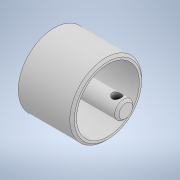
# Autodesk Inventor part: Part4
Saved by Autodesk Inventor 2021 (Build 250183000, 183)
## iProperties
Created: 2021-03-30
Part Number: Part4
Material: Generic
Document SubType Name: Modeling
Designer: Ariel Wolle
Density: 1 g/cm^3
Appearance: Default
Author: Ariel Wolle
Autodesk Inventor part; units mm, degrees
ref_plane "YZ Plane" through (0, 0, 0) normal (1, 0, 0) x (0, 1, 0)
ref_plane "XZ Plane" through (0, 0, 0) normal (0, 1, 0) x (-1, 0, 0)
ref_plane "XY Plane" through (0, 0, 0) normal (0, 0, 1) x (1, 0, 0)
sketch "Sketch1" plane through (0, 0, 0) normal (1, 0, 0) x (0, 1, 0)
  circle A0 centre (0, 0) radius 12.7
  dimension "d0" = 25.4
  constraints: 1 centre point, 1 coincident
  measures "d0" diameter of A0
extrude "Extrusion1" add sketch "Sketch1" along normal blind 19.05
sketch "Sketch2" plane through (19.05, 0, 0) normal (1, 0, 0) x (0, 0, -1)
  circle A0 centre (0, 0) radius 11.1125
  dimension "d3" = 22.225
  constraints: 1 centre point, 1 coincident
  measures "d3" diameter of A0
extrude "Extrusion2" cut sketch "Sketch2" against normal blind 15.875
sketch "Sketch3" plane through (3.175, 0, 0) normal (1, 0, 0) x (0, 0, -1)
  circle A0 centre (0, 0) radius 3.175
  dimension "d6" = 6.35
  constraints: 1 centre point, 1 coincident
  measures "d6" diameter of A0
extrude "Extrusion3" add sketch "Sketch3" along normal blind 22.225
sketch "Sketch4" plane through (0, 0, 0) normal (0, 1, 0) x (-1, 0, 0)
  circle A0 centre (-22.225, 0) radius 1.5875
  line L0 (-25.4, 3.175) -> (-25.4, -3.175) projected
  point P0 (0, 0)
  dimension "d9" = 3.175
  dimension "d10" = 3.175
  constraints: 1 centre point
  measures "d9" distance from line of L0 A0.centre
  measures "d10" diameter of A0
extrude "Extrusion4" cut sketch "Sketch4" against normal mid plane 22.225
chamfer "Chamfer1" distance 0.7937 angle 45 2 edges at (19.05, -12.7, 0) (25.4, 0, 3.175)
body "Solid1"
